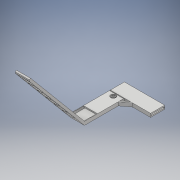
# Autodesk Inventor part: Maquinita
Saved by Autodesk Inventor 2018 (Build 220112000, 112)
## iProperties
Created: 2019-04-27
Part Number: Maquinita
Material: Genérico
Document SubType Name: Modeling
Designer: EDWIN
Density: 1 g/cm^3
Appearance: Valor por defecto
Author: EDWIN
Autodesk Inventor part; units mm, degrees
ref_plane "YZ Plane" through (0, 0, 0) normal (1, 0, 0) x (0, 1, 0)
ref_plane "XZ Plane" through (0, 0, 0) normal (0, 1, 0) x (-1, 0, 0)
ref_plane "XY Plane" through (0, 0, 0) normal (0, 0, 1) x (1, 0, 0)
sketch "Boceto1" plane through (0, 0, 0) normal (0, 0, 1) x (1, 0, 0)
  line L0 (0, 0) -> (51, 0)
  line L1 (51, 0) -> (51, 27.5)
  line L2 (51, 27.5) -> (0, 27.5)
  line L3 (-0.5, 1) -> (51, 1)
  line L4 (0, 26.5) -> (51, 26.5)
  line L5 (0, 27.5) -> (-27.5, 27.5)
  line L6 (-27.5, 27.5) -> (-27.5, -52.5)
  line L7 (-27.5, -52.5) -> (0, -52.5)
  line L8 (0, -52.5) -> (0, 0)
  line L9 (0, 26.5) -> (-26.5, 26.5)
  line L10 (-0.5, 1) -> (-1, 1)
  line L11 (-1, 1) -> (-1, -52.5)
  line L12 (-26.5, 26.5) -> (-26.5, -52.5)
  dimension "d0" = 51
  dimension "d1" = 27.5
  dimension "d2" = 1
  dimension "d3" = 1
  dimension "d4" = 27.5
  dimension "d5" = 0.5
  dimension "d6" = 1
  dimension "d7" = 1
  dimension "d8" = 80
  constraints: 26 end point, 7 perpendicular, 5 point on line, 3 horizontal, 3 parallel
  measures "d0" distance of L1.end L2.end
  measures "d1" distance of L0.end L1.end
  measures "d2" distance between parallel lines of L2 L4
  measures "d3" distance between parallel lines of L3 L0
  measures "d4" distance of L7.end L6.end
  measures "d5" distance of L3.start L10.end
  measures "d6" distance between parallel lines of L11 L8
  measures "d7" distance between parallel lines of L6 L12
  measures "d8" distance of L5.end L6.end
extrude "Extrusión1" add sketch "Boceto1" against normal blind 2.5
extrude "Extrusión2" add sketch "Boceto1" along normal blind 0.96 contours L8 L7 L11 L10 L3 L1 L0 | L4 L9 L12 L7 L6 L5 L2 L1
ref_plane "Plano de trabajo1" through (-26.5, -52.5, 0.96) normal (0, 0, 1) x (0, 1, 0)
mirror "Simetría1" about plane through (-26.5, -52.5, 0.96) normal (0, 0, 1) of "Extrusión1", "Extrusión2"
sketch "Boceto2" plane through (-27.5, 27.5, 4.42) normal (0, 0, 1) x (1, 0, 0)
  line L0 (26.5, -80) -> (26.5, -26.5) projected
  line L1 (78.5, -27.5) -> (27.5, -27.5) projected
  line L2 (26.5, -27.5) -> (0, -27.5)
  line L3 (0, -80) -> (0, 0) projected
  line L4 (27.5, -27.5) -> (27.5, -80) projected
  line L5 (26.5, -29) -> (0, -29)
  line L6 (0, -29) -> (0, -27.5)
  line L7 (26.5, -29) -> (26.5, -27.5)
  line L8 (26.5, -80) -> (26.5, -26.5) projected
  line L9 (27.5, -27.5) -> (39.5, -27.5)
  line L10 (27.5, -27.5) -> (27.5, -36.5)
  line L11 (27.5, -36.5) -> (39.5, -27.5)
  line L12 (39.5, -27.5) -> (43.5, -27.5)
  line L13 (43.5, -27.5) -> (27.5, -39.5)
  line L14 (27.5, -39.5) -> (27.5, -36.5)
  circle A0 centre (13.25, -35) radius 5
  dimension "d13" = 1.5
  dimension "d16" = 12
  dimension "d17" = 9
  dimension "d18" = 4
  dimension "d19" = 20
  dimension "d59" = 10
  dimension "d61" = 6
  constraints: 20 end point, 9 point on line, 2 horizontal, 1 centre point, 1 collinear, 1 perpendicular
  measures "d13" distance between parallel lines of L2 L5
  measures "d16" distance of L1.end L9.end
  measures "d17" distance of L1.end L10.end
  measures "d18" distance of L9.end L12.end
  measures "d19" distance of L12.end L13.end
  measures "d59" diameter of A0
  measures "d61" distance from line of L5 A0.centre
extrude "Extrusión3" cut sketch "Boceto2" against normal blind 4.42 contours L5 L3 L2 L0
extrude "Extrusión4" add sketch "Boceto2" against normal blind 6.92 contours L13 L4 L11 L1
sketch "Boceto3" plane through (-27.5, -52.5, -2.5) normal (0, -1, 0) x (1, 0, 0)
  line L0 (0, 0) -> (78.5, 0) projected
  line L1 (78.5, 2.5) -> (1, 2.5) projected
  line L2 (39.5, 6.92) -> (27.5, 6.92) projected
  line L3 (0, 6.92) -> (0, 0)
  line L4 (27.5, 0) -> (27.5, 6.92) projected
  line L5 (0, 0) -> (27.5, 0)
  line L6 (27.5, 0) -> (27.5, 6.92)
  line L7 (0, 6.92) -> (26.5, 6.92) projected
  line L8 (27.5, 6.92) -> (26.5, 6.92)
  line L9 (26.5, 2.5) -> (26.5, 4.42) projected
  line L10 (26.5, 6.92) -> (26.5, 2.5)
  line L11 (26.5, 2.5) -> (1, 2.5)
  line L12 (1, 2.5) -> (1, 4.42) projected
  line L13 (1, 2.5) -> (1, 6.92)
  line L14 (1, 6.92) -> (0, 6.92)
  constraints: 16 end point, 4 collinear, 3 perpendicular, 1 horizontal, 1 point on line
extrude "Extrusión5" add sketch "Boceto3" along normal blind 25.5 contours L3 L7 L13 L12 L1 L4 L0 | L1 L9 L10 L8 L4
sketch "Boceto4" plane through (-27.5, 27.5, -2.5) normal (-1, 0, 0) x (0, 0, 1)
  line L0 (6.92, -105.5) -> (0, -105.5) projected
  line L1 (2.5, -1) -> (2.5, -105.5) projected
  line L2 (0, 0) -> (0, -105.5) projected
  line L3 (2.5, -105.5) -> (0, -105.5)
  line L4 (0, -39.5) -> (0, -105.5) projected
  line L5 (0, -105.5) -> (127.9371, -212.852)
  line L6 (6.92, -105.5) -> (2.5, -105.5) projected
  line L7 (2.5, -105.5) -> (130.4371, -212.852)
  line L8 (6.92, -39.5) -> (6.92, -105.5) projected
  line L9 (2.5, -105.5) -> (6.92, -105.5)
  line L10 (6.92, -105.5) -> (132.2633, -210.6755)
  line L11 (127.9371, -212.852) -> (130.4371, -212.852)
  line L12 (130.4371, -212.852) -> (132.2633, -210.6755)
  point P0 (2.5, -27.5)
  point P1 (2.5, -29)
  dimension "d26" = 40
  constraints: 14 end point, 2 horizontal, 2 parallel, 1 perpendicular
  measures "d26" angle of L5 L0
extrude "Extrusión6" add sketch "Boceto4" against normal blind 27.5 contours L7 L11 L5 L0
ref_plane "Plano de trabajo2" through (-13.75, 27.5, -2.5) normal (-1, 0, 0) x (0, 0, 1)
extrude "Extrusión7" add sketch "Boceto4" against normal blind 1 contours L10 L12 L7 L0
mirror "Simetría2" about plane through (-13.75, 27.5, -2.5) normal (-1, 0, 0) of "Extrusión7"
sketch "Boceto5" plane through (-26.5, -78, 0) normal (0, 0.7660444, 0.6427876) x (1, 0, 0)
  line L0 (0, 0) -> (0, -167.01) projected
  line L1 (25.5, -167.01) -> (25.5, 0) projected
  line L2 (25.5, 0) -> (0, 0) projected
  line L3 (0, 0) -> (0, -167.01) projected
  line L4 (0, -167.01) -> (25.5, -167.01) projected
  line L5 (12.75, 0) -> (38.25, 0) construction
  circle A0 centre (12.75, -25.5) radius 10.25
  line L6 (12.75, -35.75) -> (12.75, -38.25)
  circle A1 centre (12.75, -49.25) radius 11
  line L7 (12.75, -38.25) -> (23.75, -38.25) construction
  line L8 (12.75, -60.25) -> (12.75, -62.75)
  circle A2 centre (12.75, -73.94) radius 11.19
  line L9 (12.75, -85.13) -> (12.75, -87.63)
  circle A3 centre (12.75, -99.13) radius 11.5
  line L10 (12.75, -110.63) -> (12.75, -113.13)
  circle A4 centre (12.75, -125.32) radius 12.19
  line L11 (12.75, -113.13) -> (24.94, -113.13) construction
  line L12 (12.75, -137.51) -> (12.75, -140.01)
  circle A5 centre (12.75, -152.76) radius 12.75
  line L13 (12.75, -15.25) -> (12.75, 0)
  line L14 (0, -167.01) -> (25.5, -167.01) projected
  line L15 (25.5, -167.01) -> (25.5, 0) projected
  line L16 (0, -167.01) -> (25.5, -167.01)
  line L17 (25.5, -167.01) -> (25.5, -165.51)
  line L18 (25.5, -165.51) -> (0, -165.51)
  line L19 (0, -165.51) -> (0, -167.01)
  point P0 (26.5, 50.1374)
  dimension "d37" = 22
  dimension "d41" = 22.38
  dimension "d45" = 23
  dimension "d48" = 24.38
  dimension "d35" = 20.5
  dimension "d36" = 2.5
  dimension "d40" = 2.5
  dimension "d44" = 2.5
  dimension "d47" = 2.5
  dimension "d51" = 2.5
  dimension "d53" = 25.5
  constraints: 26 end point, 8 vertical, 4 horizontal, 4 point on line, 4 vertical alignment, 2 centre point, 2 parallel, 2 point on circle, 1 midpoint, 1 perpendicular, 8 other
  measures "d35" diameter of A0
  measures "d36" distance of L6.start L6.end
  measures "d40" distance of L8.start L8.end
  measures "d44" distance of L9.start L9.end
  measures "d47" distance of L10.start L10.end
  measures "d51" distance of L12.start L12.end
  measures "d53" diameter of A5
extrude "Extrusión8" cut sketch "Boceto5" against normal through all contours A5 | A4 | A0 | A3 | A1 | A2
extrude "Extrusión9" add sketch "Boceto5" along normal blind 2.841 contours L18 L1 L4 L0
extrude "Extrusión10" cut sketch "Boceto2" against normal through all contours A0
equation "\"d59\" = sensor"
equation "\"d37\" = cincuentacen"
equation "\"d41\" = dossol"
equation "\"d45\" = veintecen"
equation "\"d48\" = cincosol"
equation "\"d35\" = diezcen"
equation "\"d53\" = UnSol"
equation "\"UnSol\" = 25.5"
equation "\"diezcen\" = 20.5"
equation "\"veintecen\" = 23"
equation "\"cincuentacen\" = 22"
equation "\"dossol\" = 22.38"
equation "\"cincosol\" = 24.38"
equation "\"sensor\" = 10"
